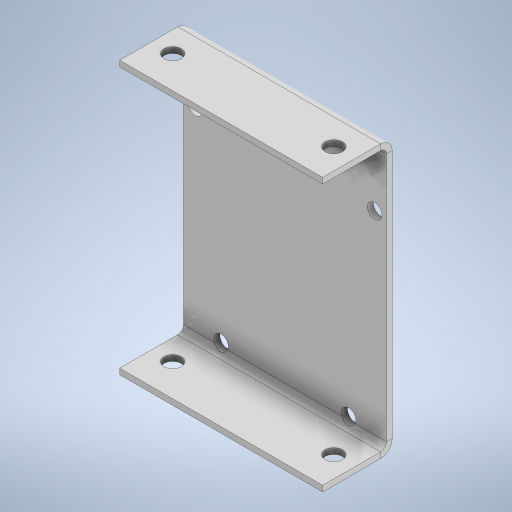
# Autodesk Inventor part: Suportmotor
Saved by Autodesk Inventor 2023 (Build 270158000, 158)
## iProperties
Created: 2022-09-23
Part Number: Suportmotor
Material: Generic
Document SubType Name: Sheet Metal
Designer: hiago.sodre
Density: 1 g/cm^3
Appearance: Default
Sheet Metal Rule: Default_mm
Author: hiago.sodre
Autodesk Inventor part; units mm, degrees
ref_plane "YZ Plane" through (0, 0, 0) normal (1, 0, 0) x (0, 1, 0)
ref_plane "XZ Plane" through (0, 0, 0) normal (0, 1, 0) x (-1, 0, 0)
ref_plane "XY Plane" through (0, 0, 0) normal (0, 0, 1) x (1, 0, 0)
sketch "Sketch12" plane through (0, 0, 0) normal (0, 0, 1) x (1, 0, 0)
  line L0 (0, 0) -> (35, 0)
  line L1 (35, 0) -> (35, 47)
  line L2 (35, 47) -> (0, 47)
  line L3 (0, 47) -> (0, 0)
  dimension "d49" = 35
  dimension "d50" = 47
  measures "d49" distance of L2.end L1.end
  measures "d50" distance of L1.end L0.end
extrude "Plate4" add sketch "Sketch12" along normal blind 1
sketch "Sketch13" plane through (0, 0, 0) normal (-1, 0, 0) x (0, 0, 1)
  point P0 (0, 0)
sketch "Sketch14" plane through (0, 46, 0) normal (0, 1, 0) x (-1, 0, 0)
  line L0 (-35, 0) -> (0, 0)
  line L1 (0, 0) -> (0, 12)
  line L2 (0, 12) -> (-35, 12)
  line L3 (-35, 12) -> (-35, 0)
  constraints: 6 end point, 1 horizontal, 1 perpendicular, 1 vertical
edge flange "Flange3" height 12 angle 90 thickness 1 bend radius 1 thickness toward (0, 1, 0) relief straight relief width 1 relief depth 0.5 edges at (17.5, 47, 1) wall of the first edge with corners at (35, 46, 0) (0, 46, 0) (0, 46, 12) (35, 46, 12)
bend "Bend3"
corner "Corner3"
sketch "Sketch15" plane through (35, 1, 0) normal (0, -1, 0) x (1, 0, 0)
  line L0 (-35, 0) -> (0, 0)
  line L1 (0, 0) -> (0, 12)
  line L2 (0, 12) -> (-35, 12)
  line L3 (-35, 12) -> (-35, 0)
  constraints: 6 end point, 1 horizontal, 1 perpendicular, 1 vertical
edge flange "Flange4" height 12 angle 90 thickness 1 bend radius 1 thickness toward (0, -1, 0) relief straight relief width 1 relief depth 0.5 edges at (17.5, 0, 1) wall of the first edge with corners at (0, 1, 0) (35, 1, 0) (35, 1, 12) (0, 1, 12)
bend "Bend4"
corner "Corner4"
sketch "Sketch16" plane through (0, 47, 12) normal (0, 1, 0) x (1, 0, 0)
  line L0 (0, 11) -> (0, 10) projected
  line L1 (0, 10) -> (0, 5.52) construction
  line L2 (0, 10) -> (0, 0) projected
  line L3 (0, 5.52) -> (3.6, 5.52) construction
  circle A0 centre (3.6, 5.52) radius 1.5
  line L4 (35, 10) -> (35, 0) projected
  line L5 (35, 10) -> (35, 5.52)
  line L6 (35, 5.52) -> (31.4, 5.52) construction
  circle A1 centre (31.4, 5.52) radius 1.5
  point P0 (0, 12)
  dimension "d72" = 4.48
  dimension "d73" = 3.6
  dimension "d74" = 3
  dimension "d75" = 4.48
  dimension "d76" = 3.6
  dimension "d77" = 3
  constraints: 8 end point, 2 centre point, 2 coincident, 2 perpendicular, 2 point on line
  measures "d72" distance of L0.end L1.end
  measures "d73" distance of L1.end L3.end
  measures "d74" diameter of A0
  measures "d75" distance of L4.start L5.end
  measures "d76" distance of L5.end L6.end
  measures "d77" diameter of A1
extrude "Extrusion4" cut sketch "Sketch16" against normal through all
sketch "Sketch17" plane through (0, 0, 1) normal (0, 0, 1) x (1, 0, 0)
  line L0 (35, 45) -> (0, 45) construction
  line L1 (0, 45) -> (2, 45) construction
  line L2 (2, 45) -> (2, 35.5) construction
  line L3 (35, 45) -> (33, 45) construction
  line L4 (33, 45) -> (33, 35.5) construction
  circle A0 centre (2, 35.5) radius 1.25
  circle A1 centre (33, 35.5) radius 1.25
  point P0 (0, 0)
  dimension "d80" = 2
  dimension "d81" = 9.5
  dimension "d82" = 2
  dimension "d83" = 2.5
  dimension "d84" = 9.5
  constraints: 8 end point, 2 centre point, 2 coincident, 2 point on line, 1 equal radius, 1 perpendicular, 1 vertical
  measures "d80" distance of L0.end L1.end
  measures "d81" distance of L1.end L2.end
  measures "d82" distance of L0.start L3.end
  measures "d83" diameter of A0
  measures "d84" distance from line of A1.centre L0
extrude "Extrusion5" cut sketch "Sketch17" against normal blind 10
sketch "Sketch18" plane through (0, 0, 1) normal (0, 0, 1) x (1, 0, 0)
  line L0 (0, 2) -> (0, 45) projected
  line L1 (0, 2) -> (6.5, 2) construction
  line L2 (6.5, 2) -> (6.5, 2.58) construction
  circle A0 centre (6.5, 2.58) radius 1.25
  line L3 (35, 45) -> (35, 2) projected
  line L4 (35, 2) -> (28.5, 2) construction
  line L5 (35, 2) -> (0, 2) projected
  line L6 (28.5, 2) -> (28.5, 2.58) construction
  circle A1 centre (28.5, 2.58) radius 1.25
  point P0 (0, 0)
  dimension "d87" = 6.5
  dimension "d88" = 0.58
  dimension "d89" = 2.5
  dimension "d90" = 6.5
  dimension "d91" = 0.58
  dimension "d92" = 2.5
  constraints: 8 end point, 2 centre point, 2 coincident, 2 perpendicular, 1 horizontal, 1 point on line
  measures "d87" distance of L0.start L1.end
  measures "d88" distance of L1.end L2.end
  measures "d89" diameter of A0
  measures "d90" distance of L3.end L4.end
  measures "d91" distance of L4.end L6.end
  measures "d92" diameter of A1
extrude "Extrusion6" cut sketch "Sketch18" against normal blind 10
sketch "Sketch20" plane through (0, 0, 1) normal (0, 0, 1) x (1, 0, 0)
  arc A0 (7.6073, 2) -> (5.3927, 2) centre (6.5, 2.58) ccw projected
  arc A1 (5.3927, 2) -> (7.6073, 2) centre (6.5, 2.58) ccw projected
  circle A2 centre (6.5, 2.58) radius 1.25
  arc A3 (29.6073, 2) -> (27.3927, 2) centre (28.5, 2.58) ccw projected
  arc A4 (27.3927, 2) -> (29.6073, 2) centre (28.5, 2.58) ccw projected
  circle A5 centre (28.5, 2.58) radius 1.25
  point P0 (0, 0)
  constraints: 2 centre point, 2 coincident, 2 concentric
extrude "Extrusion7" cut sketch "Sketch20" along normal through all
equation "\"d51\" = Thickness"
equation "\"d52\" = BendReliefWidth"
equation "\"d53\" = BendReliefDepth"
equation "\"d54\" = MinimumRemnant"
equation "\"d55\" = TransitionRadius"
equation "\"d58\" = BendRadius"
equation "\"d59\" = CornerReliefSize"
equation "\"d60\" = GapSize"
equation "\"d61\" = JacobiRadiusSize"
equation "\"d62\" = BendReliefWidth"
equation "\"d63\" = BendReliefDepth"
equation "\"d64\" = MinimumRemnant"
equation "\"d65\" = TransitionRadius"
equation "\"d68\" = BendRadius"
equation "\"d69\" = CornerReliefSize"
equation "\"d70\" = GapSize"
equation "\"d71\" = JacobiRadiusSize"
equation "\"BendRadius\" = Thickness"
equation "\"BendReliefWidth\" = Thickness"
equation "\"BendReliefDepth\" = 0.5 * Thickness"
equation "\"CornerReliefSize\" = 4 * Thickness"
equation "\"MinimumRemnant\" = 2 * Thickness"
equation "\"TransitionRadius\" = BendRadius"
equation "\"JacobiRadiusSize\" = BendRadius"
equation "\"GapSize\" = Thickness"
equation "\"Thickness\" = 1"
body "Solid3"
